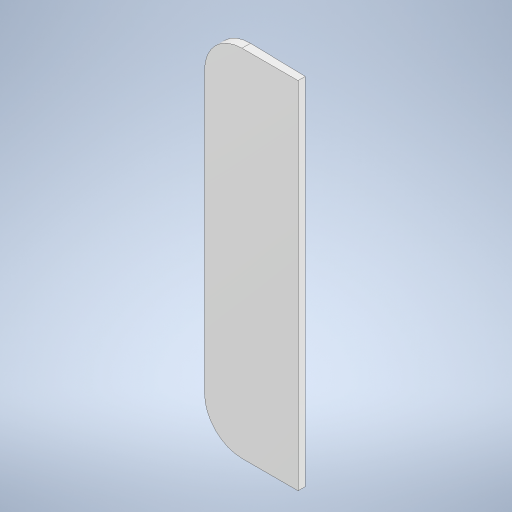
# Autodesk Inventor part: foot
Saved by Autodesk Inventor 2023 (Build 270158000, 158)
## iProperties
Created: 2022-11-05
Part Number: foot
Material: Acetalharz, Weiß
Document SubType Name: Modeling
Designer: RubenStein
Density: 1.425 g/cm^3
Appearance: Glatt - Weiß
Mass: 58.7973 g
Surface Area: 206.992 cm^2
Volume: 41.2613 cm^3
Author: RubenStein
Autodesk Inventor part; units mm, degrees
ref_plane "YZ Plane" through (0, 0, 0) normal (1, 0, 0) x (0, 1, 0)
ref_plane "XZ Plane" through (0, 0, 0) normal (0, 1, 0) x (-1, 0, 0)
ref_plane "XY Plane" through (0, 0, 0) normal (0, 0, 1) x (1, 0, 0)
sketch "Skizze1" plane through (0, 0, 0) normal (0, 1, 0) x (-1, 0, 0)
  line L0 (0, 0) -> (0, -5)
  line L1 (0, -5) -> (-50, -3.8636)
  line L2 (-50, -3.8636) -> (-50, 0)
  line L3 (-50, 0) -> (0, 0)
  line L4 (0, -5) -> (-220, 0) construction
  dimension "d2" = 5
  dimension "d3" = 50
  dimension "d4" = 0
  dimension "d5" = 220
  constraints: 10 end point, 1 collinear, 1 parallel, 1 perpendicular, 1 vertical
  measures "d2" distance of L0.start L0.end
  measures "d3" distance of L2.end L0.start
  measures "d4" vertical distance of L4.end L0.start
  measures "d5" distance of L4.end L0.start
extrude "Extrusion1" add sketch "Skizze1" along normal blind 190
fillet "Rundung1" radius 20 2 edges at (0, 190, -2.5) (0, 0, -2.5)
